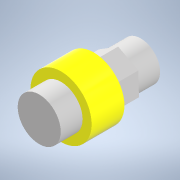
# Autodesk Inventor part: SC DC MOTOR
Saved by Autodesk Inventor 2021 (Build 250183000, 183)
## iProperties
Created: 2021-07-25
Part Number: SC DC MOTOR
Material: Generic
Document SubType Name: Modeling
Designer: HP
Density: 1 g/cm^3
Appearance: Default
Author: HP
Autodesk Inventor part; units mm, degrees
ref_plane "YZ Plane" through (0, 0, 0) normal (1, 0, 0) x (0, 1, 0)
ref_plane "XZ Plane" through (0, 0, 0) normal (0, 1, 0) x (-1, 0, 0)
ref_plane "XY Plane" through (0, 0, 0) normal (0, 0, 1) x (1, 0, 0)
sketch "Sketch1" plane through (0, 0, 0) normal (0, 0, 1) x (1, 0, 0)
  circle A0 centre (0, 0) radius 2.2451
  constraints: 1 centre point, 1 coincident
extrude "Extrusion1" add sketch "Sketch1" against normal blind 5.08
sketch "Sketch2" plane through (0, 0, 0) normal (0, 0, 1) x (1, 0, 0)
  circle A0 centre (0, 0) radius 2.2451 projected
  line L0 (2.2451, 1.3979) -> (2.3331, -1.2453)
  line L1 (2.3331, -1.2453) -> (0.0881, -2.6432)
  line L2 (0.0881, -2.6432) -> (-2.2451, -1.3979)
  line L3 (-2.2451, -1.3979) -> (-2.3331, 1.2453)
  line L4 (-2.3331, 1.2453) -> (-0.0881, 2.6432)
  line L5 (-0.0881, 2.6432) -> (2.2451, 1.3979)
  constraints: 12 end point, 1 coincident, 13 other
extrude "Extrusion2" add sketch "Sketch2" along normal blind 0.381 and the other way blind 2.54 contours A0 | L0 L1 L2 L3 L4 L5
sketch "Sketch3" plane through (0, 0, 0.381) normal (0, 0, 1) x (1, 0, 0)
  circle A0 centre (0, 0) radius 3.5571
  constraints: 1 centre point, 1 coincident
extrude "Extrusion3" add sketch "Sketch3" along normal blind 3.81
sketch "Sketch4" plane through (0, 0, 4.191) normal (0, 0, 1) x (1, 0, 0)
  circle A0 centre (0, 0) radius 2.5038
  constraints: 1 centre point, 1 coincident
extrude "Extrusion4" add sketch "Sketch4" along normal blind 2.54
body "Solid1"
